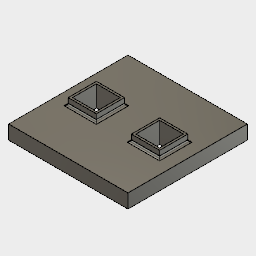
base (Autodesk Fusion 360 design; units mm, degrees)
Autodesk Fusion 360 part; units mm, degrees
sketch "Sketch1" plane through (0, 0, 0) normal (0, 1, 0) x (1, 0, 0)
  line L0 (0, -85) -> (85, -85)
  line L1 (85, -85) -> (85, 85)
  line L2 (85, 85) -> (-85, 85)
  line L3 (-85, 85) -> (-85, -85)
  line L4 (-85, -85) -> (0, -85)
  dimension "d4" = 170
  dimension "d5" = 170
  measures "d4" distance of L1.end L2.end
  measures "d5" distance of L2.end L3.end
extrude "Extrude1" add sketch "Sketch1" along normal blind 20
sketch "Sketch2" plane through (0, 20, 0) normal (0, 1, 0) x (-1, 0, 0)
  line L0 (85, 85) -> (-85, 85)
  line L1 (-85, 85) -> (-85, -85)
  line L2 (-85, -85) -> (85, -85)
  line L3 (85, -85) -> (85, 85)
  line L4 (65, 0) -> (65, -20)
  line L5 (65, -20) -> (25, -20)
  line L6 (25, -20) -> (25, 20)
  line L7 (25, 20) -> (65, 20)
  line L8 (65, 20) -> (65, 0)
  line L9 (-25, 0) -> (-25, -20)
  line L10 (-25, -20) -> (-65, -20)
  line L11 (-65, -20) -> (-65, 20)
  line L12 (-65, 20) -> (-25, 20)
  line L13 (-25, 20) -> (-25, 0)
  dimension "d13" = 40
  dimension "d14" = 40
  dimension "d17" = 40
  dimension "d18" = 40
  measures "d13" distance of L4.end L5.end
  measures "d14" distance of L5.end L6.end
  measures "d17" distance of L9.end L10.end
  measures "d18" distance of L10.end L11.end
extrude "Extrude2" add sketch "Sketch2" along normal blind 10 contours L4 L5 L6 L7 L8 | L9 L10 L11 L12 L13
sketch "Sketch3" plane through (0, 30, 0) normal (0, 1, 0) x (-1, 0, 0)
  line L0 (-25, 20) -> (-65, 20)
  line L1 (-65, 20) -> (-65, -20)
  line L2 (-65, -20) -> (-25, -20)
  line L3 (-25, -20) -> (-25, 20)
  line L4 (-28, 0) -> (-28, -17)
  line L5 (-28, -17) -> (-62, -17)
  line L6 (-62, -17) -> (-62, 17)
  line L7 (-62, 17) -> (-28, 17)
  line L8 (-28, 17) -> (-28, 0)
  dimension "d24" = 34
  dimension "d25" = 34
  measures "d24" distance of L4.end L5.end
  measures "d25" distance of L5.end L6.end
extrude "Extrude3" cut sketch "Sketch3" against normal blind 50 contours L4 L5 L6 L7 L8
sketch "Sketch4" plane through (0, 30, 0) normal (0, 1, 0) x (-1, 0, 0)
  line L0 (65, 20) -> (25, 20)
  line L1 (25, 20) -> (25, -20)
  line L2 (25, -20) -> (65, -20)
  line L3 (65, -20) -> (65, 20)
  line L4 (62, 0) -> (62, -17)
  line L5 (62, -17) -> (28, -17)
  line L6 (28, -17) -> (28, 17)
  line L7 (28, 17) -> (62, 17)
  line L8 (62, 17) -> (62, 0)
  dimension "d31" = 34
  dimension "d32" = 34
  measures "d31" distance of L4.end L5.end
  measures "d32" distance of L5.end L6.end
extrude "Extrude4" cut sketch "Sketch4" against normal blind 50 contours L4 L5 L6 L7 L8
fillet "Fillet1" radius 3 1 edges at (-45, 20, 20)
fillet "Fillet2" radius 3 1 edges at (-25, 20, 1.5)
fillet "Fillet3" radius 3 1 edges at (45, 20, 20)
fillet "Fillet4" radius 3 1 edges at (65, 20, 1.5)
fillet "Fillet5" radius 3 4 edges at (25, 20, 1.5) (46.5, 20, -20) (-43.5, 20, -20) (-65, 20, 1.5)
